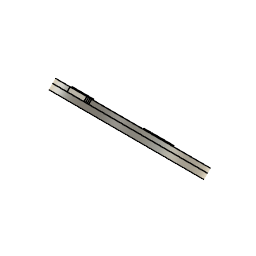
Fed Insert (Autodesk Fusion 360 design; units mm, degrees)
Autodesk Fusion 360 part; units mm, degrees
other "Base Mesh Feature1"
other "Modify1"
sketch "Well Side Plane" plane through (8.9061, 0, 0) normal (1, 0, 0) x (0, 1, 0)
  line L0 (30.1961, 26.2144) -> (24.5763, 31.8874)
  line L1 (23.8335, 31.1501) -> (17.7877, 37.198)
  line L2 (-7.9854, 62.9728) -> (0.9552, 54.0298)
  line L3 (-13.6839, 70.0914) -> (-7.2456, 63.7109)
other "MeshSection3"
sketch "Well Front Plane" plane through (0, 6.9805, 0) normal (0, 1, 0) x (-1, 0, 0)
  line L0 (-31.2383, 49.4201) -> (-36.9498, 49.4084)
  line L1 (-18.0262, 47.9831) -> (-31.2974, 47.9448)
  line L2 (0.1222, 48.0303) -> (13.5729, 48.0673)
  line L3 (13.4961, 49.5426) -> (19.3041, 49.5591)
other "MeshSection4"
ref_plane "WorkPlane1" through (31.2383, 6.9805, 49.4201) normal (-0.001935, -0.707194, -0.707017) x (0.999996, -0.002737, 0)
ref_plane "WorkPlane2" through (31.2381, 6.9097, 49.3494) normal (-0.001935, -0.707194, -0.707017) x (0.999996, -0.002737, 0)
sketch "Sketch7" plane through (31.2383, 6.9805, 49.4201) normal (-0.001935, -0.707194, -0.707017) x (0.999996, -0.002737, 0)
  circle A0 centre (-22.2973, -1.7567) radius 31.0134
  circle A1 centre (-22.3808, -2.2949) radius 22.4979
  circle A2 centre (-4.6149, -9.8198) radius 4.6309
  circle A3 centre (-39.9628, -9.819) radius 4.6304
other "MeshSection6"
sketch "Sketch11" plane through (31.2381, 6.9097, 49.3494) normal (-0.001935, -0.707194, -0.707017) x (0.999996, -0.002737, 0)
  ellipse E0 centre (-25.7359, 23.7749) end of major axis (-29.7024, 23.6237) minor radius 3.5061
other "MeshSection8"
sketch "Sketch9" plane through (0.0773, 28.2438, 28.2368) normal (-0.001935, -0.707194, -0.707017) x (0.999996, -0.002737, 0)
  circle A0 centre (8.9217, 28.1973) radius 31.0134 construction
  line L0 (8.9217, -2.8161) -> (8.9217, 59.2107) construction
  line L1 (22.8684, 3.7059) -> (27.1216, 3.7059)
  line L2 (-5.0249, 3.7059) -> (-9.2782, 3.7059)
  arc A1 (-5.0249, 3.7059) -> (22.8684, 3.7059) centre (8.9217, 28.1973) ccw
  arc A2 (27.1216, 3.7059) -> (-9.2782, 3.7059) centre (8.9217, 28.1973) ccw
  circle A3 centre (8.9217, 28.1973) radius 3
  ellipse E0 centre (5.4831, 53.7289) end of major axis (1.5167, 53.5777) minor radius 3.5061
  ellipse E1 centre (5.4831, 53.7289) end of major axis (1.017, 53.5586) minor radius 4.0061
  dimension "d4" = 6
  constraint coincident A0 L0.start
  constraint coincident A0 L0.end
  constraint vertical L0
  constraint horizontal L1
  constraint perpendicular L0 L2
  constraint concentric A0 A1
  constraint concentric A0 A2
  constraint concentric A1 A3
  measures "d4" diameter of A3
extrude "Extrude1" add sketch "Sketch9" along normal blind -0.5 and the other way blind -2 contours L1 L2 A1 A2 makes body 1
sketch "Sketch12" plane through (0.0783, 28.5974, 28.5903) normal (0.001935, 0.707194, 0.707017) x (-0.999996, 0.002737, 0)
  circle A0 centre (-8.9217, 28.1973) radius 3
  ellipse E0 centre (-5.4831, 53.7289) end of major axis (-1.017, 53.5586) minor radius 4.0061
  arc A1 (-22.8684, 3.7059) -> (5.0249, 3.7059) centre (-8.9217, 28.1973) ccw
  line L0 (5.0249, 3.7059) -> (9.2782, 3.7059)
  arc A2 (9.2782, 3.7059) -> (-27.1216, 3.7059) centre (-8.9217, 28.1973) ccw
  line L1 (-27.1216, 3.7059) -> (-22.8684, 3.7059)
  circle A3 centre (8.7438, 20.135) radius 4.6304
  circle A4 centre (-26.6042, 20.1342) radius 4.6309
extrude "Extrude2" cut sketch "Sketch12" against normal blind 3.2 draft -45 contours A3 | A4 bodies 1
sketch "Sketch1" plane through (0.0783, 28.5974, 28.5903) normal (0.001935, 0.707194, 0.707017) x (-0.999996, 0.002737, 0) in component "Cut Template"
  circle A0 centre (-26.6042, 20.1342) radius 4.6309
  circle A1 centre (8.7438, 20.135) radius 4.6304
  ellipse E0 centre (-5.4831, 53.7289) end of major axis (-1.017, 53.5586) minor radius 4.0061
  circle A2 centre (-8.9217, 28.1973) radius 3
  arc A3 (-22.8684, 3.7059) -> (5.0249, 3.7059) centre (-8.9217, 28.1973) ccw
  line L0 (5.0249, 3.7059) -> (9.2782, 3.7059)
  arc A4 (9.2782, 3.7059) -> (-27.1216, 3.7059) centre (-8.9217, 28.1973) ccw
  line L1 (-27.1216, 3.7059) -> (-22.8684, 3.7059)
  arc A5 (9.2782, 3.7059) -> (-27.1216, 3.7059) centre (-8.9217, 28.1973) ccw
  line L2 (-27.1216, 3.7059) -> (-22.8684, 3.7059)
  line L3 (5.0249, 3.7059) -> (9.2782, 3.7059)
  arc A6 (-22.8684, 3.7059) -> (5.0249, 3.7059) centre (-8.9217, 28.1973) ccw
  circle A7 centre (8.7438, 20.135) radius 4.6304 construction
  circle A8 centre (-26.6042, 20.1342) radius 4.6309 construction
  circle A9 centre (-8.9217, 28.1973) radius 3 construction
  ellipse E1 centre (-5.4831, 53.7289) end of major axis (-1.017, 53.5586) minor radius 4.0061
  line L4 (-20.7998, 17.3616) -> (-28.3169, 13.9338)
  line L5 (-29.3767, 14.3298) -> (-32.8045, 21.8469)
  line L6 (-32.4085, 22.9067) -> (-24.8914, 26.3345)
  line L7 (-23.8316, 25.9385) -> (-20.4038, 18.4214)
  line L8 (-20.0719, 17.6935) -> (-33.1364, 22.5748) construction
  line L9 (-29.0448, 13.6019) -> (-24.1635, 26.6664) construction
  line L10 (-8.9217, 28.1973) -> (-8.9217, 0.0133)
  line L11 (-29.0448, 13.6019) -> (-34.2742, 11.2174) construction
  line L12 (-33.1364, 22.5748) -> (-38.3658, 20.1903) construction
  line L13 (-6.2709, 24.7465) -> (-11.5725, 24.7465)
  line L14 (-12.3725, 25.5465) -> (-12.3725, 30.8481)
  line L15 (-11.5725, 31.6481) -> (-6.2709, 31.6481)
  line L16 (-5.4709, 30.8481) -> (-5.4709, 25.5465)
  line L17 (-5.4709, 24.7465) -> (-12.3725, 31.6481) construction
  line L18 (-12.3725, 24.7465) -> (-5.4709, 31.6481) construction
  line L19 (-8.9217, 28.1973) -> (-4.8489, 58.4376) construction
  line L20 (-8.9217, 28.1973) -> (-10.137, 49.7194) construction
  line L21 (-8.9217, 28.1973) -> (-2.0558, 48.631) construction
  line L22 (-6.0964, 49.1752) -> (-2.8632, 48.7398)
  line L23 (-6.0964, 49.1752) -> (-9.3296, 49.6107)
  line L24 (-10.1829, 50.5328) -> (-10.6419, 58.6622)
  line L25 (-1.7963, 49.4033) -> (0.7971, 57.1215)
  circle A10 centre (-8.9217, 8.2463) radius 4.5
  circle A11 centre (8.3563, 38.1728) radius 4.5
  circle A12 centre (-26.1998, 38.1728) radius 4.5
  line L26 (-28.3169, 13.9338) -> (-27.902, 13.024)
  line L27 (-28.6299, 12.6921) -> (-29.0448, 13.6019)
  arc A13 (-28.6299, 12.6921) -> (-27.902, 13.024) centre (-28.266, 12.858) ccw
  line L28 (-12.3725, 23.7465) -> (-12.3725, 24.7465)
  arc A14 (-12.3725, 23.7465) -> (-11.5725, 23.7465) centre (-11.9725, 23.7465) ccw
  line L29 (-11.5725, 24.7465) -> (-11.5725, 23.7465)
  line L30 (-10.0806, 48.721) -> (-10.137, 49.7194)
  line L31 (-9.3296, 49.6107) -> (-9.2819, 48.7661)
  arc A15 (-10.0806, 48.721) -> (-9.2819, 48.7661) centre (-9.6812, 48.7435) ccw
  line L32 (-29.9547, 13.187) -> (-29.0448, 13.6019)
  arc A16 (-30.2866, 13.9149) -> (-29.9547, 13.187) centre (-30.1206, 13.551) ccw
  line L33 (-29.3767, 14.3298) -> (-30.2866, 13.9149)
  line L34 (-20.7998, 17.3616) -> (-20.3849, 16.4517)
  arc A17 (-20.3849, 16.4517) -> (-19.657, 16.7837) centre (-20.021, 16.6177) ccw
  line L35 (-19.657, 16.7837) -> (-20.0719, 17.6935)
  line L36 (-19.1621, 18.1084) -> (-20.0719, 17.6935)
  arc A18 (-19.1621, 18.1084) -> (-19.494, 18.8363) centre (-19.328, 18.4724) ccw
  line L37 (-20.4038, 18.4214) -> (-19.494, 18.8363)
  line L38 (-23.8316, 25.9385) -> (-22.9217, 26.3534)
  arc A19 (-22.9217, 26.3534) -> (-23.2537, 27.0813) centre (-23.0877, 26.7174) ccw
  line L39 (-23.2537, 27.0813) -> (-24.1635, 26.6664)
  line L40 (-24.5784, 27.5763) -> (-24.1635, 26.6664)
  arc A20 (-24.5784, 27.5763) -> (-25.3063, 27.2444) centre (-24.9424, 27.4103) ccw
  line L41 (-24.8914, 26.3345) -> (-25.3063, 27.2444)
  line L42 (-32.4085, 22.9067) -> (-32.8234, 23.8166)
  arc A21 (-32.8234, 23.8166) -> (-33.5513, 23.4847) centre (-33.1874, 23.6506) ccw
  line L43 (-33.5513, 23.4847) -> (-33.1364, 22.5748)
  line L44 (-34.0463, 22.1599) -> (-33.1364, 22.5748)
  arc A22 (-34.0463, 22.1599) -> (-33.7144, 21.432) centre (-33.8803, 21.796) ccw
  line L45 (-32.8045, 21.8469) -> (-33.7144, 21.432)
  line L46 (14.5651, 22.9067) -> (7.048, 26.3345)
  line L47 (14.5651, 22.9067) -> (14.98, 23.8166)
  arc A23 (15.7079, 23.4847) -> (14.98, 23.8166) centre (15.344, 23.6506) ccw
  line L48 (15.7079, 23.4847) -> (15.293, 22.5748)
  line L49 (16.2029, 22.1599) -> (15.293, 22.5748)
  arc A24 (15.871, 21.432) -> (16.2029, 22.1599) centre (16.0369, 21.796) ccw
  line L50 (14.9611, 21.8469) -> (15.871, 21.432)
  line L51 (11.5333, 14.3298) -> (14.9611, 21.8469)
  line L52 (11.5333, 14.3298) -> (12.4432, 13.9149)
  arc A25 (12.1113, 13.187) -> (12.4432, 13.9149) centre (12.2772, 13.551) ccw
  line L53 (12.1113, 13.187) -> (11.2014, 13.6019)
  line L54 (10.7865, 12.6921) -> (11.2014, 13.6019)
  arc A26 (10.0586, 13.024) -> (10.7865, 12.6921) centre (10.4226, 12.858) ccw
  line L55 (10.4735, 13.9338) -> (10.0586, 13.024)
  line L56 (2.9564, 17.3616) -> (10.4735, 13.9338)
  line L57 (2.9564, 17.3616) -> (2.5415, 16.4517)
  arc A27 (1.8136, 16.7837) -> (2.5415, 16.4517) centre (2.1775, 16.6177) ccw
  line L58 (1.8136, 16.7837) -> (2.2285, 17.6935)
  line L59 (1.3186, 18.1084) -> (2.2285, 17.6935)
  arc A28 (1.6505, 18.8363) -> (1.3186, 18.1084) centre (1.4846, 18.4724) ccw
  line L60 (2.5604, 18.4214) -> (1.6505, 18.8363)
  line L61 (5.9882, 25.9385) -> (2.5604, 18.4214)
  line L62 (5.9882, 25.9385) -> (5.0783, 26.3534)
  arc A29 (5.4102, 27.0813) -> (5.0783, 26.3534) centre (5.2443, 26.7174) ccw
  line L63 (5.4102, 27.0813) -> (6.3201, 26.6664)
  line L64 (6.735, 27.5763) -> (6.3201, 26.6664)
  arc A30 (7.4629, 27.2444) -> (6.735, 27.5763) centre (7.099, 27.4103) ccw
  line L65 (7.048, 26.3345) -> (7.4629, 27.2444)
  arc A31 (-13.3725, 25.5465) -> (-13.3725, 24.7465) centre (-13.3725, 25.1465) ccw
  line L66 (-12.3725, 25.5465) -> (-13.3725, 25.5465)
  line L67 (-13.3725, 24.7465) -> (-12.3725, 24.7465)
  line L68 (-6.2709, 24.7465) -> (-6.2709, 23.7465)
  arc A32 (-6.2709, 23.7465) -> (-5.4709, 23.7465) centre (-5.8709, 23.7465) ccw
  line L69 (-5.4709, 23.7465) -> (-5.4709, 24.7465)
  line L70 (-4.4709, 24.7465) -> (-5.4709, 24.7465)
  arc A33 (-4.4709, 24.7465) -> (-4.4709, 25.5465) centre (-4.4709, 25.1465) ccw
  line L71 (-5.4709, 25.5465) -> (-4.4709, 25.5465)
  line L72 (-5.4709, 30.8481) -> (-4.4709, 30.8481)
  arc A34 (-4.4709, 30.8481) -> (-4.4709, 31.6481) centre (-4.4709, 31.2481) ccw
  line L73 (-4.4709, 31.6481) -> (-5.4709, 31.6481)
  line L74 (-5.4709, 32.6481) -> (-5.4709, 31.6481)
  arc A35 (-5.4709, 32.6481) -> (-6.2709, 32.6481) centre (-5.8709, 32.6481) ccw
  line L75 (-6.2709, 31.6481) -> (-6.2709, 32.6481)
  line L76 (-11.5725, 31.6481) -> (-11.5725, 32.6481)
  arc A36 (-11.5725, 32.6481) -> (-12.3725, 32.6481) centre (-11.9725, 32.6481) ccw
  line L77 (-12.3725, 32.6481) -> (-12.3725, 31.6481)
  line L78 (-13.3725, 31.6481) -> (-12.3725, 31.6481)
  arc A37 (-13.3725, 31.6481) -> (-13.3725, 30.8481) centre (-13.3725, 31.2481) ccw
  line L79 (-12.3725, 30.8481) -> (-13.3725, 30.8481)
  line L80 (-10.9708, 50.6389) -> (-10.1829, 50.5328)
  arc A38 (-10.9708, 50.6389) -> (-11.0578, 49.8434) centre (-11.0243, 50.2423) ccw
  line L81 (-10.137, 49.7194) -> (-11.0578, 49.8434)
  line L82 (-1.0084, 49.2972) -> (-1.7963, 49.4033)
  arc A39 (-1.135, 48.507) -> (-1.0084, 49.2972) centre (-1.0618, 48.9005) ccw
  line L83 (-2.0558, 48.631) -> (-1.135, 48.507)
  line L84 (-2.3743, 47.6831) -> (-2.0558, 48.631)
  arc A40 (-3.1326, 47.9379) -> (-2.3743, 47.6831) centre (-2.7535, 47.8105) ccw
  line L85 (-2.8632, 48.7398) -> (-3.1326, 47.9379)
  line L86 (-10.0806, 48.721) -> (-9.2819, 48.7661) construction
  point P0 (-26.6042, 20.1342)
  point P1 (-8.9217, 28.1973)
  dimension "d17" = 0.3
  dimension "d19" = 0.3
  dimension "d20" = 9
  dimension "d22" = 360
  dimension "d27" = 0.8
  dimension "d28" = 1
  dimension "d29" = 0.8
  dimension "d30" = 1
  dimension "d32" = 1
  dimension "d34" = 360
  dimension "d36" = 360
  dimension "d39" = 0.8
  dimension "d40" = 0.8
  constraint perpendicular L4 L5
  constraint parallel L4 L6
  constraint parallel L5 L7
  constraint coincident L8 P0
  constraint coincident L9 P0
  constraint coincident P0 A0.centre
  constraint coincident P1 A2.centre
  constraint midpoint A6 L10.end
  constraint coincident A5 L11.end
  constraint perpendicular L5 L11
  constraint coincident A5 L12.end
  constraint perpendicular L5 L12
  constraint equal L11 L12
  constraint horizontal L13
  constraint perpendicular L13 L14
  constraint parallel L13 L15
  constraint parallel L14 L16
  constraint coincident L17 P1
  constraint coincident L18 P1
  constraint coincident E0.centre L19
  constraint coincident A5 L19.end
  constraint symmetric L19 P1 A2.centre
  constraint coincident L19 L22.start
  constraint perpendicular L19 L22
  constraint perpendicular L19 L23
  constraint coincident A5 L24.end
  constraint parallel L20 L24
  constraint coincident A5 L25.end
  constraint parallel L21 L25
  constraint coincident L10 A10.centre
  constraint tangent L27 A13
  constraint tangent L28 A14
  constraint coincident L18.start L28.end
  constraint vertical L28
  constraint vertical L29
  constraint equal L28 L29
  constraint tangent L30 A15
  constraint coincident L20.end L30.end
  constraint symmetric L11.start L9 L27.end
  constraint symmetric L9 L4.end L5.start
  constraint symmetric L9 L26.end A16.start
  constraint symmetric L9 L27.start L32.start
  constraint symmetric L9 A13 A16
  constraint symmetric L9.start L10 L53.end
  constraint symmetric L10 L4.end L55.start
  constraint symmetric L10 L26.end A26.start
  constraint symmetric L10 L27.start L54.start
  constraint symmetric L10 A13 A26
  constraint symmetric L10 L32.start A25.start
  constraint symmetric L10 L9.start L53.end
  constraint symmetric L10 A16.start L52.end
  constraint symmetric L10 A16 A25
  constraint symmetric L10 L5.start L51.start
  constraint symmetric L10 L4.start L56.start
  constraint symmetric L10 L34.end L57.end
  constraint symmetric L10 A17.end A27.start
  constraint symmetric L10 A17 A27
  constraint symmetric L10 L8.start L58.end
  constraint symmetric L10 L36.start L59.start
  constraint symmetric L10 A18.end A28.start
  constraint symmetric L10 A18 A28
  constraint symmetric L10 L7.end L60.start
  constraint symmetric L10 L7.start L61.start
  constraint symmetric L10 L38.end L62.end
  constraint symmetric L10 A19.end A29.start
  constraint symmetric L10 A19 A29
  constraint symmetric L10 L9.end L63.end
  constraint symmetric L10 L40.start L64.start
  constraint symmetric L10 A20.end A30.start
  constraint symmetric L10 A20 A30
  constraint symmetric L10 L6.end L46.end
  constraint symmetric L10 L6.start L46.start
  constraint symmetric L10 L42.end L47.end
  constraint symmetric L10 A21.end A23.start
  constraint symmetric L10 A21 A23
  constraint symmetric L10 L8.end L48.end
  constraint symmetric L10 L44.start L49.start
  constraint symmetric L10 A22.end A24.start
  constraint symmetric L10 A22 A24
  constraint symmetric L10 L5.end L50.start
  constraint symmetric L18 A14.end A31.start
  constraint symmetric L18 L28.start A31.end
  constraint symmetric L18 L13.end L14.start
  constraint symmetric L18 A14 A31
  constraint symmetric L18 L28.end L67.end
  constraint tangent L80 A38
  constraint collinear L23 L81
  constraint parallel L80 L81
  constraint symmetric L19 L20.end L21.end
  constraint symmetric L19 L31.end A40.start
  constraint symmetric L19 L30.start L84.start
  constraint symmetric L19 L23.end L22.end
  constraint symmetric L19 A15 A40
  constraint symmetric L19 L80.start L82.start
  constraint symmetric L19 A38.end A39.start
  constraint symmetric L19 A38 A39
  constraint symmetric L19 L24.start L25.start
  constraint collinear L24 L30
  constraint parallel L30 L31
  constraint coincident A15.centre L86
  measures "d17" distance of A8 L6
  measures "d19" distance of A0 L7
  measures "d20" diameter of A10
  measures "d27" distance of L9.start L4.end
  measures "d28" distance of L9.start L27.start
  measures "d29" distance of L18.start L13.end
  measures "d30" distance of L18.start L28.start
  measures "d32" distance of L20.end L30.start
  measures "d39" distance of L80 L81
  measures "d40" distance of L20 L31
extrude "Extrude1'" add sketch "Sketch1" along normal blind 2 separate body contours A3 L0 A4 L1 A5 L2 L3 A6 L22 L23 L24 L25 L30 L31 A15 L80 A38 L81 L82 A39 L83 L84 A40 L85 | L10 A10 | L10 A10 | A11 | A12 makes body 2 in component "Cut Template"
extrude "Extrude2'" add sketch "Sketch1" along normal blind 0.4 from surface at 2 contours L10 A10 | L10 A10 | A11 | A12 bodies 2 in component "Cut Template"
mesh_step "MeshTessellate1"
mesh_step "MeshCombine1"
other "MeshRepair2"
component "Cut Template" placed x (1, 0, 0) y (0, 1, 0) z (0, 0, 1) at (0, 0, 0)
